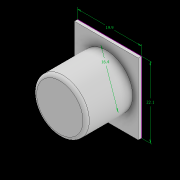
# Autodesk Inventor part: LV-MaxSonar-EZ
Saved by Autodesk Inventor 2022 (Build 260153000, 153)
## iProperties
Created: 2021-09-27
Part Number: LV-MaxSonar-EZ
Material: Genérico
Document SubType Name: Modeling
Designer: Julio R
Density: 1 g/cm^3
Appearance: Valor por defecto
Author: Julio R
Autodesk Inventor part; units mm, degrees
ref_plane "YZ Plane" through (0, 0, 0) normal (1, 0, 0) x (0, 1, 0)
ref_plane "XZ Plane" through (0, 0, 0) normal (0, 1, 0) x (-1, 0, 0)
ref_plane "XY Plane" through (0, 0, 0) normal (0, 0, 1) x (1, 0, 0)
sketch "Boceto1" plane through (0, 0, 0) normal (0, 0, 1) x (1, 0, 0)
  line L0 (0, 0) -> (19.9, 0)
  line L1 (19.9, 0) -> (19.9, 22.1)
  line L2 (19.9, 22.1) -> (0, 22.1)
  line L3 (0, 22.1) -> (0, 0)
  circle A0 centre (9.95, 11.05) radius 8.2
  dimension "d0" = 19.9
  dimension "d1" = 22.1
  dimension "d2" = 16.4
  constraints: 8 end point, 2 parallel, 1 centre point, 1 horizontal, 1 perpendicular
  measures "d0" distance of L2.end L1.end
  measures "d1" distance of L1.end L0.end
  measures "d2" diameter of A0
extrude "Extrusión1" add sketch "Boceto1" along normal blind 1
extrude "Extrusión2" add sketch "Boceto1" along normal blind 15.5 contours A0
fillet "Empalme1" radius 1 1 edges at (1.75, 11.05, 15.5)
